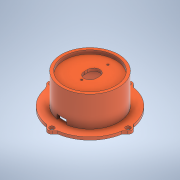
# Autodesk Inventor part: sombreronuevasversionsanti
Saved by Autodesk Inventor 2021 (Build 250183000, 183)
## iProperties
Created: 2021-04-01
Part Number: sombreronuevasversionsanti
Material: Genérico
Document SubType Name: Modeling
Designer: Arturo
Density: 1 g/cm^3
Appearance: Valor por defecto
Author: Arturo
Autodesk Inventor part; units mm, degrees
ref_plane "YZ Plane" through (0, 0, 0) normal (1, 0, 0) x (0, 1, 0)
ref_plane "XZ Plane" through (0, 0, 0) normal (0, 1, 0) x (-1, 0, 0)
ref_plane "XY Plane" through (0, 0, 0) normal (0, 0, 1) x (1, 0, 0)
sketch "Boceto1" plane through (0, 0, 0) normal (0, 1, 0) x (-1, 0, 0)
  line L0 (0, 0) -> (12.5, 0)
  line L1 (12.5, 0) -> (12.5, 5)
  line L2 (12.5, 5) -> (0, 5)
  line L3 (0, 5) -> (0, 0)
  circle A0 centre (6.25, 2.5) radius 1
  arc A1 (8.4861, 0) -> (4.0139, 0) centre (6.25, -2) ccw
  circle A2 centre (6.25, -25) radius 1
  line L4 (6.25, -25) -> (6.25, -22.5)
  line L5 (0, -22.5) -> (12.5, -22.5)
  line L6 (12.5, -22.5) -> (12.5, -27.5)
  line L7 (12.5, -27.5) -> (0, -27.5)
  line L8 (0, -27.5) -> (0, -22.5)
  line L9 (6.25, 0) -> (6.25, -6.25)
  arc A3 (12.5, -6.25) -> (0, -6.25) centre (6.25, -6.25) ccw
  arc A4 (0, -10.25) -> (12.5, -10.25) centre (6.25, -10.25) ccw
  line L10 (12.5, -10.25) -> (12.5, -6.25)
  line L11 (0, -10.25) -> (0, -6.25)
  circle A5 centre (6.25, -6.25) radius 27
  circle A6 centre (6.25, -6.25) radius 30
  dimension "d0" = 12.5
  dimension "d1" = 5
  dimension "d2" = 2
  dimension "d4" = 6
  dimension "d6" = 2
  dimension "d7" = 2.5
  dimension "d8" = 12.5
  dimension "d9" = 5
  dimension "d10" = 6.25
  dimension "d11" = 12.5
  dimension "d13" = 12.5
  dimension "d14" = 54
  dimension "d15" = 60
  constraints: 24 end point, 7 centre point, 6 point on circle, 4 parallel, 4 tangent, 3 coincident, 2 horizontal, 2 perpendicular, 2 point on line, 1 midpoint, 1 vertical
  measures "d0" distance of L2.end L1.end
  measures "d1" distance of L1.end L0.end
  measures "d2" diameter of A0
  measures "d4" diameter of A1
  measures "d6" diameter of A2
  measures "d7" distance of L4.start L4.end
  measures "d8" distance of L6.end L7.end
  measures "d9" distance of L5.end L6.end
  measures "d10" distance of L9.start L9.end
  measures "d11" diameter of A3
  measures "d13" diameter of A4
  measures "d14" diameter of A5
  measures "d15" diameter of A6
extrude "Extrusión1" add sketch "Boceto1" along normal blind 3 contours A5
extrude "Extrusión2" add sketch "Boceto1" along normal blind 6.8 contours A6
extrude "Extrusión3" add sketch "Boceto1" against normal blind 5 contours L3 L2 L1 L0 A1 | L5 L6 L7 L8
sketch "Boceto2" plane through (0, 0, 0) normal (0, 1, 0) x (1, 0, 0)
  line L0 (-4.0139, 0) -> (0, 0) projected
  arc A0 (-8.4861, 0) -> (-4.0139, 0) centre (-6.25, 2) ccw projected
  line L1 (-12.5, 0) -> (-8.4861, 0) projected
  line L2 (-12.5, -5) -> (-12.5, 0) projected
  line L3 (0, -5) -> (-12.5, -5) projected
  line L4 (0, 0) -> (0, -5) projected
  circle A1 centre (-6.25, -2.5) radius 1 projected
  line L5 (0, 27.5) -> (0, 22.5) projected
  line L6 (-12.5, 27.5) -> (0, 27.5) projected
  line L7 (-12.5, 22.5) -> (-12.5, 27.5) projected
  line L8 (0, 22.5) -> (-12.5, 22.5) projected
  circle A2 centre (-6.25, 25) radius 1 projected
  line L9 (-12.5, -5) -> (-12.5, 0) projected
  line L10 (-6.25, 0) -> (0, 0) projected
  line L11 (-12.5, -5) -> (0, -5)
  line L12 (0, -5) -> (0, 0)
  line L13 (-12.5, 0) -> (-12.5, -5)
  line L14 (-12.5, 27.5) -> (0, 27.5) projected
  line L15 (0, 22.5) -> (-12.5, 22.5) projected
  line L16 (0, 27.5) -> (-12.5, 27.5)
  line L17 (-12.5, 27.5) -> (-12.5, 22.5)
  line L18 (-12.5, 22.5) -> (0, 22.5)
  line L19 (0, 22.5) -> (0, 27.5)
  circle A3 centre (-6.25, -2.5) radius 1
  circle A4 centre (-6.25, 25) radius 1
  arc A5 (-8.4861, 0) -> (-4.0139, 0) centre (-6.25, 2) ccw
  line L20 (0, 0) -> (-4.0139, 0)
  line L21 (-8.4861, 0) -> (-12.5, 0)
  line L22 (-8.4861, 0) -> (-4.0139, 0)
  point P0 (-8.4861, 0)
  dimension "d22" = 2
  dimension "d23" = 2
  dimension "d24" = 6
  constraints: 20 end point, 5 parallel, 3 centre point, 3 coincident, 3 horizontal, 2 perpendicular, 2 point on circle
  measures "d22" diameter of A3
  measures "d23" diameter of A4
  measures "d24" diameter of A5
extrude "Extrusión4" add sketch "Boceto2" along normal blind 3
sketch "Boceto3" plane through (-6.25, 0, -6.25) normal (0, -1, 0) x (1, 0, 0)
  circle A0 centre (0, 0) radius 30
  circle A1 centre (0, 0) radius 27
  point P0 (6.25, 6.25)
  dimension "d27" = 60
  dimension "d28" = 54
  constraints: 2 centre point, 1 coincident
  measures "d27" diameter of A0
  measures "d28" diameter of A1
extrude "Extrusión5" add sketch "Boceto3" along normal blind 25
sketch "Boceto4" plane through (-6.25, -25, -6.25) normal (0, -1, 0) x (1, 0, 0)
  circle A0 centre (0, 0) radius 30
  circle A1 centre (0, 0) radius 27
  circle A2 centre (0, 40) radius 2.5
  arc A3 (3.3493, 42.1868) -> (-3.3436, 42.1955) centre (0, 40) ccw
  circle A4 centre (40, 0) radius 2.5
  arc A5 (42.2251, -3.324) -> (42.295, 3.2761) centre (40, 0) ccw
  circle A6 centre (0, -40) radius 2.5
  arc A7 (-3.111, -42.5143) -> (3.3503, -42.1853) centre (0, -40) ccw
  circle A8 centre (-40, 0) radius 2.5
  arc A9 (-42.5143, 3.111) -> (-42.5143, -3.111) centre (-40, 0) ccw
  line L0 (-3.995, 39.8) -> (-3.995, 39.8)
  arc A10 (3.3493, 42.1868) -> (5.8327, 39.5725) centre (11.7225, 47.6539) ccw
  arc A11 (-5.8604, 39.5684) -> (-3.3436, 42.1955) centre (-11.7026, 47.6843) ccw
  arc A12 (39.5114, 6.2326) -> (5.8327, 39.5725) centre (0, 0) ccw
  arc A13 (5.8279, -39.5732) -> (39.5535, -5.9597) centre (0, 0) ccw
  arc A14 (-5.8604, 39.5684) -> (-39.04, 8.7108) centre (0, 0) ccw
  arc A15 (-39.04, -8.7108) -> (-8.7108, -39.04) centre (0, 0) ccw
  line L1 (-3.995, -39.8) -> (-6.9108, -38.8236)
  line L2 (8.3455, -38.2373) -> (8.1717, -38.2997)
  arc A16 (42.2251, -3.324) -> (39.5535, -5.9597) centre (47.7877, -11.6341) ccw
  arc A17 (39.5114, 6.2326) -> (42.295, 3.2761) centre (48.0324, 11.4665) ccw
  arc A18 (5.8279, -39.5732) -> (3.3503, -42.1853) centre (11.726, -47.6486) ccw
  arc A19 (-3.111, -42.5143) -> (-8.7108, -39.04) centre (-10.8885, -48.8) ccw
  arc A20 (-42.5143, 3.111) -> (-39.04, 8.7108) centre (-48.8, 10.8885) ccw
  arc A21 (-39.04, -8.7108) -> (-42.5143, -3.111) centre (-48.8, -10.8885) ccw
  point P0 (6.25, 6.25)
  dimension "d32" = 60
  dimension "d33" = 54
  dimension "d34" = 5
  dimension "d35" = 8
  dimension "d36" = 5
  dimension "d37" = 8
  dimension "d38" = 5
  dimension "d39" = 8
  dimension "d40" = 5
  dimension "d41" = 8
  dimension "d42" = 10
  dimension "d43" = 10
  constraints: 35 point on circle, 22 centre point, 12 tangent, 6 end point, 6 equal radius, 5 coincident
  measures "d32" diameter of A0
  measures "d33" diameter of A1
  measures "d34" diameter of A2
  measures "d35" diameter of A3
  measures "d36" diameter of A4
  measures "d37" diameter of A5
  measures "d38" diameter of A6
  measures "d39" diameter of A7
  measures "d40" diameter of A8
  measures "d41" diameter of A9
  measures "d42" radius of A10
  measures "d43" radius of A16
extrude "Extrusión6" add sketch "Boceto4" along normal blind 3 contours A0 | A10 A12 A17 A5 A16 A13 A18 A7 A19 A15 A21 A9 A20 A14 A11 A3
sketch "Boceto5" plane through (0, 0, 0) normal (0, 0, 1) x (1, 0, 0)
  line L0 (-2.9007, -25) -> (-9.5936, -25) projected
  line L1 (-9.5936, -25) -> (-9.5936, -28) projected
  line L2 (-2.9007, -28) -> (-9.5936, -28) projected
  line L3 (-2.9007, -25) -> (-2.9007, -28) projected
  line L4 (-9.5936, -25) -> (-12.1104, -25) projected
  line L5 (-12.1104, -25) -> (-12.1104, -28) projected
  line L6 (-9.5936, -28) -> (-12.1104, -28) projected
  line L7 (-9.5936, -25) -> (-9.5936, -28) projected
  line L8 (-0.4173, -25) -> (-2.9007, -25) projected
  line L9 (-2.9007, -25) -> (-2.9007, -28) projected
  line L10 (-0.4173, -28) -> (-2.9007, -28) projected
  line L11 (-0.4173, -25) -> (-0.4173, -28) projected
  line L12 (-6.2472, -25) -> (-1.2472, -25)
  line L13 (-0.4173, -25) -> (-2.9007, -25) projected
  line L14 (-1.2472, -25) -> (-11.2472, -25)
  line L15 (-11.2472, -25) -> (-1.2472, -25)
  line L16 (-1.2472, -25) -> (-1.2472, -20)
  line L17 (-1.2472, -20) -> (-11.2472, -20)
  line L18 (-11.2472, -20) -> (-11.2472, -25)
  point P0 (0, 0)
  dimension "d46" = 5
  dimension "d47" = 10
  dimension "d48" = 10
  dimension "d49" = 5
  constraints: 12 end point, 2 parallel, 2 point on line, 1 horizontal, 1 midpoint, 1 perpendicular
  measures "d46" distance of L12.start L12.end
  measures "d47" distance of L12.end L14.end
  measures "d48" distance of L17.end L16.end
  measures "d49" distance of L16.end L15.end
extrude "Extrusión7" cut sketch "Boceto5" along normal blind 40 contours L0 L4 L18 L17 L16 L8
